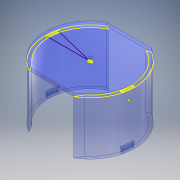
# Autodesk Inventor part: Gear Container V2
Saved by Autodesk Inventor 2017 (Build 210142000, 142)
## iProperties
Created: 2019-01-21
Part Number: Gear Container V2
Material: Generic
Document SubType Name: Modeling
Designer: Matt
Density: 1 g/cm^3
Appearance: Clear - Blue
Author: Matt
Autodesk Inventor part; units mm, degrees
ref_plane "YZ Plane" through (0, 0, 0) normal (1, 0, 0) x (0, 1, 0)
ref_plane "XZ Plane" through (0, 0, 0) normal (0, 1, 0) x (-1, 0, 0)
ref_plane "XY Plane" through (0, 0, 0) normal (0, 0, 1) x (1, 0, 0)
sketch "Sketch1" plane through (0, 0, 0) normal (0, 0, 1) x (1, 0, 0)
  circle A0 centre (0, 0) radius 63.25
  circle A1 centre (0, 0) radius 68.25
  dimension "d0" = 126.5
  dimension "d1" = 5
  constraints: 2 centre point, 1 coincident
  measures "d0" diameter of A0
  measures "d1" radial gap between concentric circles of A0 A1
extrude "Extrusion1" add sketch "Sketch1" along normal blind 81.2
sketch "Sketch2" plane through (0, 0, 81.2) normal (0, 0, 1) x (1, 0, 0)
  circle A0 centre (0, 0) radius 68.25
  constraints: 1 centre point, 1 coincident
extrude "Extrusion2" add sketch "Sketch2" along normal blind 5
sketch "Sketch3" plane through (0, 0, 86.2) normal (0, 0, 1) x (1, 0, 0)
  circle A0 centre (0, 0) radius 2.75
  dimension "d6" = 5.5
  constraints: 1 centre point, 1 coincident
  measures "d6" diameter of A0
extrude "Extrusion3" cut sketch "Sketch3" against normal blind 5
sketch "Sketch4" plane through (0, 0, 86.2) normal (0, 0, 1) x (1, 0, 0)
  line L0 (0, 0) -> (-34.125, 59.1062)
  circle A0 centre (0, 0) radius 68.25 projected
  line L1 (0, 0) -> (68.25, 0) construction
  circle A1 centre (0, 0) radius 2.75 projected
  line L2 (0, 0) -> (34.125, 59.1062)
  line L3 (34.125, 59.1062) -> (-34.125, 59.1062)
  line L4 (0, 0) -> (-34.125, -59.1062)
  circle A2 centre (0, 0) radius 68.25 projected
  line L5 (0, 0) -> (68.25, 0) construction
  line L6 (0, 0) -> (34.125, -59.1062)
  line L7 (0, 0) -> (68.25, 0) construction
  line L8 (34.125, -59.1062) -> (-34.125, -59.1062)
  dimension "d9" = 120
  dimension "d15" = 120
  dimension "d16" = 60
  constraints: 18 end point, 4 point on circle, 3 equal length, 3 horizontal
  measures "d9" angle of L1 L0
  measures "d15" angle of L4 L5
  measures "d16" angle of L6 L7
extrude "Extrusion4" cut sketch "Sketch4" against normal through all contours A0 L3 | L8 A0
sketch "Sketch5" plane through (0, 0, 0) normal (0, 0, -1) x (-1, 0, 0)
  line L0 (-34.125, 59.1062) -> (34.125, 59.1062) projected
  line L1 (34.125, 59.1062) -> (28.4813, 56.4746)
  arc A0 (-22.517, 59.1062) -> (22.517, 59.1062) centre (0, 0) ccw projected
  line L2 (34.125, 59.1062) -> (40.3521, 59.1062) construction
  line L3 (0, 0) -> (0, 13.3987)
  line L4 (-34.125, 59.1062) -> (-28.4813, 56.4746)
  arc A1 (-22.517, 59.1062) -> (-28.4813, 56.4746) centre (0, 0) ccw
  line L5 (-34.125, 59.1062) -> (-22.517, 59.1062)
  dimension "d12" = 155
  constraints: 10 end point, 3 point on circle, 2 horizontal, 1 centre point, 1 concentric, 1 equal length, 1 point on line, 1 symmetric about line, 1 vertical
  measures "d12" angle of L1 L2
extrude "Extrusion5" cut sketch "Sketch5" against normal blind 81.2 contours L0 A0 L4 | L0 L1 A0
sketch "Sketch6" plane through (-34.125, 59.1062, 86.2) normal (0, 1, 0) x (1, 0, 0)
  point P0 (34.125, 86.2)
sketch "Sketch7" plane through (0, 0, 0) normal (0, 0, -1) x (-1, 0, 0)
  arc A0 (34.125, -59.1062) -> (34.125, 59.1062) centre (0, 0) ccw projected
  line L0 (34.125, 59.1062) -> (28.4813, 56.4746) projected
  arc A1 (22.517, -59.1062) -> (28.4813, 56.4746) centre (0, 0) ccw projected
  line L1 (22.517, -59.1062) -> (34.125, -59.1062) projected
  arc A2 (34.125, -59.1062) -> (34.125, 59.1062) centre (0, 0) ccw projected
  line L2 (-28.4813, 56.4746) -> (-34.125, 59.1062) projected
  arc A3 (-34.125, 59.1062) -> (-34.125, -59.1062) centre (0, 0) ccw projected
  line L3 (-34.125, -59.1062) -> (-22.517, -59.1062) projected
  arc A4 (-28.4813, 56.4746) -> (-22.517, -59.1062) centre (0, 0) ccw projected
  line L4 (22.517, -59.1062) -> (34.125, -59.1062) projected
  line L5 (34.125, -59.1062) -> (39.929, -49.0534)
  arc A5 (22.517, -59.1062) -> (28.4813, 56.4746) centre (0, 0) ccw projected
  line L6 (34.125, -59.1062) -> (45.733, -59.1062) construction
  circle A6 centre (0, 0) radius 2.75 projected
  line L7 (0, 0) -> (0, -7.8217)
  line L8 (-34.125, -59.1062) -> (-39.929, -49.0534)
  line L9 (34.125, -59.1062) -> (22.517, -59.1062)
  arc A7 (22.517, -59.1062) -> (39.929, -49.0534) centre (0, 0) ccw
  line L10 (34.125, -59.1062) -> (39.929, -49.0534)
  dimension "d17" = 60
  constraints: 12 end point, 3 point on circle, 2 horizontal, 2 symmetric about line, 1 centre point, 1 equal length, 1 vertical
  measures "d17" angle of L6 L5
extrude "Extrusion6" cut sketch "Sketch7" against normal blind 81.2 contours L1 A1 L5
mirror "Mirror1" about plane through (0, 0, 0) normal (1, 0, 0) of "Extrusion6"
sketch "Sketch8" plane through (0, 0, 0) normal (0, 0, -1) x (-1, 0, 0)
  arc A0 (39.929, -49.0534) -> (28.4813, 56.4746) centre (0, 0) ccw projected
  line L0 (63.25, 0) -> (68.25, 0)
  arc A1 (34.125, -59.1062) -> (34.125, 59.1062) centre (0, 0) ccw projected
  arc A2 (64.25, 0) -> (67.25, 0) centre (65.75, 0) ccw
  line L1 (61.4481, 14.99) -> (66.3056, 16.1749)
  arc A3 (65.3341, 15.9379) -> (62.4196, 15.227) centre (63.8768, 15.5825) ccw
  arc A4 (67.25, 0) -> (65.3341, 15.9379) centre (-0.9999, -0.1202) ccw
  arc A5 (64.25, 0) -> (62.4196, 15.227) centre (-3.9983, -0.4806) ccw
  line L2 (0, 0) -> (0, 7.6651)
  line L3 (0, 0) -> (-11.2866, 0)
  arc A6 (-64.25, 0) -> (-62.4196, -15.227) centre (3.9983, 0.4806) ccw
  arc A7 (-65.3341, -15.9379) -> (-62.4196, -15.227) centre (-63.8768, -15.5825) ccw
  arc A8 (-67.25, 0) -> (-65.3341, -15.9379) centre (0.9999, 0.1202) ccw
  arc A9 (-64.25, 0) -> (-67.25, 0) centre (-65.75, 0) ccw
  dimension "d20" = 3
  dimension "d21" = 5
  dimension "d22" = 3
  dimension "d23" = 68.25
  dimension "d24" = 68.25
  constraints: 28 point on circle, 8 centre point, 8 end point, 4 point on line, 4 symmetric about line, 2 horizontal, 2 midpoint, 1 vertical
  measures "d20" diameter of A2
  measures "d21" distance of L1.start L1.end
  measures "d22" diameter of A3
  measures "d23" radius of A4
  measures "d24" radius of A5
extrude "Extrusion7" cut sketch "Sketch8" against normal blind 8 contours A5 L1 A4 L0 | L0 A2 | A3 L1 | A6 A7 A8 A9
sketch "Sketch9" plane through (0, 0, 0) normal (0, 0, -1) x (-1, 0, 0)
  arc A0 (64.25, 0) -> (67.25, 0) centre (65.75, 0) ccw projected
  arc A1 (64.75, 0) -> (66.75, -0.0027) centre (65.75, 0) ccw
  arc A2 (64.8496, 15.8142) -> (64.8483, 15.8195) centre (63.8768, 15.5825) ccw
  arc A3 (64.75, 0) -> (63.1516, 14.2694) centre (-3.4987, -0.4206) ccw
  line L0 (0, 0) -> (0, 7.6651) projected
  circle A4 centre (0, 0) radius 2.75 projected
  line L1 (34.125, -59.1062) -> (-34.125, -59.1062) projected
  line L2 (39.929, -49.0534) -> (34.125, -59.1062) projected
  arc A5 (39.929, -49.0534) -> (28.4813, 56.4746) centre (0, 0) ccw projected
  line L3 (34.125, 59.1062) -> (28.4813, 56.4746) projected
  line L4 (-34.125, 59.1062) -> (34.125, 59.1062) projected
  line L5 (-28.4813, 56.4746) -> (-34.125, 59.1062) projected
  arc A6 (-28.4813, 56.4746) -> (-39.929, -49.0534) centre (0, 0) ccw projected
  line L6 (-39.929, -49.0534) -> (-34.125, -59.1062) projected
  line L7 (0, 0) -> (-11.2866, 0) projected
  arc A7 (64.25, 0) -> (62.4196, 15.227) centre (-3.9983, -0.4806) ccw projected
  arc A8 (67.25, 0) -> (65.3341, 15.9379) centre (-0.9999, -0.1202) ccw projected
  arc A9 (64.25, 0) -> (67.25, 0) centre (65.75, 0) ccw projected
  arc A10 (-64.75, 0) -> (-66.75, -0.0027) centre (-65.75, 0) ccw
  arc A11 (-65.1039, -14.7194) -> (-65.3397, -15.9149) centre (-63.877, -15.5823) ccw
  arc A12 (-64.849, -15.8165) -> (-64.849, -15.8165) centre (-63.8765, -15.5834) ccw
  arc A13 (-64.25, 0) -> (-62.4196, -15.227) centre (3.9983, 0.4806) ccw
  arc A14 (-64.75, 0) -> (-63.1534, -14.2595) centre (3.4986, 0.4224) ccw
  arc A15 (-66.75, -0.0027) -> (-65.1039, -14.7194) centre (1.4998, 0.1807) ccw
  arc A16 (-67.25, 0) -> (-65.3341, -15.9379) centre (0.9999, 0.1202) ccw
  arc A17 (-64.25, 0) -> (-67.25, 0) centre (-65.75, 0) ccw
  arc A18 (-64.75, 0) -> (-66.75, -0.0027) centre (-65.75, 0) ccw
  arc A19 (66.75, -0.0027) -> (65.1039, 14.7197) centre (-1.4998, -0.1803) ccw
  arc A20 (64.8496, 15.8142) -> (64.8483, 15.8195) centre (-1.4998, -0.1803) ccw
  arc A21 (-67.25, 0) -> (-66.7377, -1.1289) centre (-65.75, 0) ccw
  arc A22 (-64.7342, -1.1037) -> (-64.25, 0) centre (-65.75, 0) ccw
  arc A23 (65.1039, 14.7197) -> (65.3341, 15.9379) centre (63.8768, 15.5825) ccw
  arc A24 (62.4196, 15.227) -> (63.1516, 14.2694) centre (63.8768, 15.5825) ccw
  arc A25 (-65.3341, -15.9379) -> (-65.3341, -15.9379) centre (-63.877, -15.5823) ccw
  arc A26 (-62.4196, -15.227) -> (-63.1534, -14.2595) centre (-63.8795, -15.5722) ccw
  point P0 (65.3341, 15.9379)
  dimension "d28" = 2
  dimension "d30" = 68.25
  constraints: 56 point on circle, 20 centre point, 8 symmetric about line, 6 coincident, 1 tangent, 2 other
  measures "d28" diameter of A2
  measures "d30" radius of A3
extrude "Extrusion8" add sketch "Sketch9" against normal blind 4 contours A7 A24 A3 A1 A19 A23 A8 A0 | A21 A15 A11 A16 | A10 A15 A21 A17 A22 A14 | A22 A13 A26 A14
sketch "Sketch10" plane through (0, 0, 81.2) normal (0, 0, -1) x (-1, 0, 0)
  point P0 (0, 0)
sketch "Sketch11" plane through (0, 0, 81.2) normal (0, 0, -1) x (-1, 0, 0)
  arc A0 (-65.3397, -15.9149) -> (-65.3341, -15.9379) centre (0.9999, 0.1202) ccw projected
  arc A1 (-65.1039, -14.7194) -> (-65.3397, -15.9149) centre (-63.877, -15.5823) ccw projected
  arc A2 (-66.75, -0.0027) -> (-65.1039, -14.7194) centre (1.4998, 0.1807) ccw projected
  arc A3 (-64.75, 0) -> (-66.75, -0.0027) centre (-65.75, 0) ccw projected
  arc A4 (-64.75, 0) -> (-63.1534, -14.2595) centre (3.4986, 0.4224) ccw projected
  arc A5 (-62.4196, -15.227) -> (-63.1534, -14.2595) centre (-63.8795, -15.5722) ccw projected
  arc A6 (-65.3341, -15.9379) -> (-62.4196, -15.227) centre (-63.8768, -15.5825) ccw projected
  line L0 (-34.125, -59.1062) -> (-39.929, -49.0534) projected
  arc A7 (-28.4813, 56.4746) -> (-39.929, -49.0534) centre (0, 0) ccw projected
  line L1 (-28.4813, 56.4746) -> (-34.125, 59.1062) projected
  arc A8 (-34.125, 59.1062) -> (-34.125, -59.1062) centre (0, 0) ccw projected
  arc A9 (65.1039, 14.7197) -> (63.1516, 14.2694) centre (63.8768, 15.5825) ccw projected
  arc A10 (66.75, -0.0027) -> (65.1039, 14.7197) centre (-1.4998, -0.1803) ccw projected
  arc A11 (64.75, 0) -> (66.75, -0.0027) centre (65.75, 0) ccw projected
  arc A12 (64.75, 0) -> (63.1516, 14.2694) centre (-3.4987, -0.4206) ccw projected
  line L2 (39.929, -49.0534) -> (34.125, -59.1062) projected
  arc A13 (34.125, -59.1062) -> (34.125, 59.1062) centre (0, 0) ccw projected
  line L3 (34.125, 59.1062) -> (28.4813, 56.4746) projected
  arc A14 (39.929, -49.0534) -> (28.4813, 56.4746) centre (0, 0) ccw projected
  circle A15 centre (0, 0) radius 2.75 projected
  line L4 (0, 0) -> (65.75, 0)
  line L5 (0, 0) -> (63.8768, 15.5825)
  constraints: 4 end point, 1 horizontal
body "Solid1"
